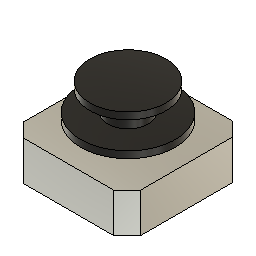
Aspen Hand Support Medium v6 (Autodesk Fusion 360 archive; units mm, degrees)
design "Mini 2 Axis Analog Thumbstick-2765"
Autodesk Fusion 360 part; units mm, degrees
sketch "Sketch1" plane through (0, 0, 0) normal (0, 0, 1) x (1, 0, 0)
  line L0 (8.65, -8.775) -> (-8.65, -8.775)
  line L1 (-8.65, -8.775) -> (-8.65, 8.775)
  line L2 (-8.65, 8.775) -> (8.65, 8.775)
  line L3 (8.65, 8.775) -> (8.65, -8.775)
  line L4 (8.65, -8.775) -> (-8.65, 8.775) construction
  line L5 (-8.65, -8.775) -> (8.65, 8.775) construction
  dimension "d1" = 17.3
  dimension "d2" = 17.55
  constraint horizontal L0
  constraint perpendicular L0 L1
  constraint parallel L0 L2
  constraint parallel L1 L3
  constraint coincident L4 origin
  constraint coincident L5 origin
  measures "d1" distance of L1.end L2.end
  measures "d2" distance of L0.start L2.end
extrude "Extrude1" add sketch "Sketch1" along normal blind 5.8 makes body 1
chamfer "Chamfer1" distance 2 angle 45 4 edges at (8.65, -8.775, 2.9) (-8.65, -8.775, 2.9) (-8.65, 8.775, 2.9) (8.65, 8.775, 2.9) on bodies 1
sketch "Sketch3" plane through (0, 0, 5.8) normal (0, 0, 1) x (-1, 0, 0)
  line L0 (-8.65, -6.775) -> (-6.65, -8.775)
  line L1 (-6.65, -8.775) -> (6.65, -8.775)
  line L2 (6.65, -8.775) -> (8.65, -6.775)
  line L3 (8.65, -6.775) -> (8.65, 6.775)
  line L4 (8.65, 6.775) -> (6.65, 8.775)
  line L5 (6.65, 8.775) -> (-6.65, 8.775)
  line L6 (-6.65, 8.775) -> (-8.65, 6.775)
  line L7 (-8.65, 6.775) -> (-8.65, -6.775)
  circle A0 centre (0, 0) radius 4.1
  dimension "d6" = 8.2
  constraint coincident A0.centre origin
  measures "d6" diameter of A0
extrude "Extrude2" cut sketch "Sketch3" against normal blind 0.3 contours A0 bodies 1
sketch "Sketch4" plane through (0, 0, 5.5) normal (0, 0, 1) x (-1, 0, 0)
  circle A0 centre (0, 0) radius 4.1
  line L0 (-0.525, -1.475) -> (0.525, -1.475)
  arc A1 (0.525, -1.475) -> (0.525, 1.475) centre (0.525, 0) ccw
  line L1 (0.525, 1.475) -> (-0.525, 1.475)
  arc A2 (-0.525, 1.475) -> (-0.525, -1.475) centre (-0.525, 0) ccw
  line L2 (-0.525, 0) -> (0.525, 0) construction
  dimension "d9" = 2.95
  dimension "d10" = 1.05
  constraint tangent L0 A1
  constraint tangent A1 L1
  constraint parallel L0 L1
  constraint tangent L1 A2
  constraint tangent L0 A2
  constraint horizontal L2
  constraint coincident A0.centre origin
  constraint midpoint L2 A0.centre
  measures "d9" diameter of A1
  measures "d10" distance of A2.centre A1.centre
extrude "Extrude3" add sketch "Sketch4" along normal blind 4.04 contours L0 A1 L1 A2 bodies 1
sketch "Sketch1 (2)" plane through (0, 0, 0) normal (0, 0, 1) x (1, 0, 0) in component "Standard Topper"
  circle A0 centre (0, 0) radius 6.95
  dimension "d13" = 13.9
  constraint coincident A0.centre origin
  measures "d13" diameter of A0
extrude "Extrude1'" add sketch "Sketch1 (2)" along normal blind 1 separate body makes body 2 in component "Standard Topper"
copy_body "Body->Comp1" bodies 1 removing the originals makes body 3 in component "Joystick Base"
sketch "Sketch3 (2)" plane through (0, 0, 1) normal (0, 0, 1) x (-1, 0, 0) in component "Standard Topper"
  circle A0 centre (0, 0) radius 6.95
  circle A1 centre (0, 0) radius 3
  dimension "d17" = 6
  constraint coincident A0.centre A1.centre
  measures "d17" diameter of A1
extrude "Extrude2'" add sketch "Sketch3 (2)" along normal blind 3 contours A1 bodies 2 in component "Standard Topper"
sketch "Sketch4 (2)" plane through (0, 0, 4) normal (0, 0, 1) x (-1, 0, 0) in component "Standard Topper"
  circle A0 centre (0, 0) radius 3
  circle A1 centre (0, 0) radius 5.6
  dimension "d20" = 11.2
  constraint coincident A0.centre A1.centre
  measures "d20" diameter of A1
extrude "Extrude3'" add sketch "Sketch4 (2)" along normal blind 1 contours A0 | A1 bodies 2 in component "Standard Topper"
sketch "Sketch5" plane through (0, 0, 0) normal (0, 0, -1) x (1, 0, 0) in component "Standard Topper"
  circle A0 centre (0, 0) radius 6.95
  line L0 (-0.5, -1.5) -> (0.5, -1.5)
  arc A1 (0.5, -1.5) -> (0.5, 1.5) centre (0.5, 0) ccw
  line L1 (0.5, 1.5) -> (-0.5, 1.5)
  arc A2 (-0.5, 1.5) -> (-0.5, -1.5) centre (-0.5, 0) ccw
  line L2 (-0.5, 0) -> (0.5, 0) construction
  constraint tangent L0 A1
  constraint tangent A1 L1
  constraint parallel L0 L1
  constraint tangent L1 A2
  constraint tangent L0 A2
  constraint horizontal L2
  constraint coincident A0.centre origin
  constraint midpoint L2 A0.centre
extrude "Extrude4" cut sketch "Sketch5" against normal blind 2.54 contours L0 A1 L1 A2 bodies 2 in component "Standard Topper"
sketch "Sketch1 (3)" plane through (-5.9469, -8.775, -11.757) normal (0, -1, 0) x (1, 0, 0) in component "Joystick Base"
  line L0 (-0.7031, 17.557) -> (-0.7031, 11.757)
  line L1 (-0.7031, 11.757) -> (12.5969, 11.757)
  line L2 (12.5969, 11.757) -> (12.5969, 17.557)
  line L3 (12.5969, 17.557) -> (-0.7031, 17.557)
  line L4 (5.5569, 12.007) -> (6.3369, 12.007)
  line L5 (6.3369, 12.007) -> (6.3369, 8.407)
  line L6 (6.3369, 8.407) -> (5.5569, 8.407)
  line L7 (5.5569, 8.407) -> (5.5569, 12.007)
  dimension "d33" = 0.78
  dimension "d34" = 3.6
  dimension "d35" = 0.25
  dimension "d36" = 6.26
  constraint horizontal L4
  constraint vertical L5
  constraint horizontal L6
  constraint vertical L7
  measures "d33" distance of L5.end L6.end
  measures "d34" distance of L4.end L5.end
  measures "d35" distance of L1 L4
  measures "d36" distance of L0 L7
extrude "Extrude1''" [suppressed] in component "Joystick Base"
pattern_linear "R-Pattern1" [suppressed] in component "Joystick Base"
sketch "Sketch2" plane through (8.65, 0.6667, 1.3826) normal (1, 0, 0) x (0, 1, 0) in component "Joystick Base"
  line L0 (6.1083, -1.3826) -> (6.1083, 4.4174)
  line L1 (6.1083, 4.4174) -> (-7.4417, 4.4174)
  line L2 (-7.4417, 4.4174) -> (-7.4417, -1.3826)
  line L3 (-7.4417, -1.3826) -> (6.1083, -1.3826)
component "Standard Topper" placed x (1, 0, 0) y (0, 1, 0) z (0, 0, 1) at (0, 0, 7)
component "Joystick Base" placed x (1, 0, 0) y (0, 1, 0) z (0, 0, 1) at (0, 0, 0)
equation "d11 = 4.3 mm - 0.26 mm"

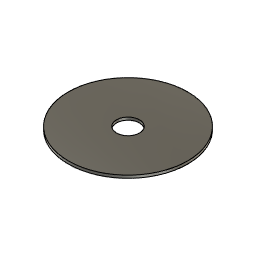
design "Inner cover disk"
Autodesk Fusion 360 part; units mm, degrees
sketch "Sketch1" plane through (0, 0, 0) normal (0, 0, 1) x (1, 0, 0)
  circle A0 centre (0, 0) radius 2.5
  circle A1 centre (0, 0) radius 13
  dimension "d1" = 26
  constraint coincident A0.centre A1.centre
  constraint concentric A0 A1
  measures "d1" diameter of A1
extrude "Extrude1" add sketch "Sketch1" along normal blind 0.6
